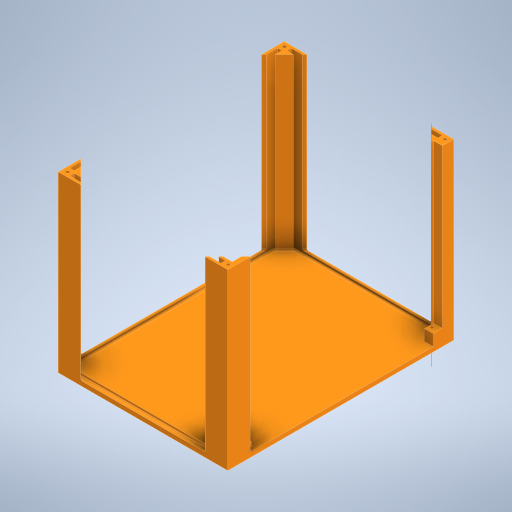
# Autodesk Inventor part: Cabinet
Saved by Autodesk Inventor 2024.3 (Build 283343000, 343)
## iProperties
Created: 2025-03-25
Part Number: Cabinet
Material: Všeobecné
Document SubType Name: Modeling
Designer: admin
Density: 1 g/cm^3
Appearance: Oranžová
Author: admin
Autodesk Inventor part; units mm, degrees
ref_plane "YZ Plane" through (0, 0, 0) normal (1, 0, 0) x (0, 1, 0)
ref_plane "XZ Plane" through (0, 0, 0) normal (0, 1, 0) x (-1, 0, 0)
sketch "Náčrt1" plane through (0, 0, 0) normal (0, 1, 0) x (-1, 0, 0)
  line L0 (75, 100) -> (-75, 100)
  line L1 (-75, 100) -> (-75, -100)
  line L2 (-75, -100) -> (75, -100)
  line L3 (75, -100) -> (75, 100)
  line L4 (105, 0) -> (-105, 0) projected
  line L5 (0, -140) -> (0, 140) projected
  point P0 (0, 0)
  dimension "d0" = 200
  dimension "d1" = 150
  constraints: 8 end point, 2 parallel, 1 horizontal, 1 perpendicular, 2 other
  measures "d0" distance of L2.end L0.start
  measures "d1" distance of L0.start L0.end
extrude "Vysunutí1" add sketch "Náčrt1" along normal blind 4
sketch "Náčrt2" plane through (0, 4, 0) normal (0, 1, 0) x (1, 0, 0)
  line L0 (-75, -100) -> (-75, -80)
  line L1 (-75, -100) -> (-55, -100)
  line L2 (-75, 100) -> (-75, -100) projected
  line L3 (-75, -100) -> (75, -100) projected
  line L4 (-69, -86) -> (-69, -92)
  line L5 (-69, -92) -> (-73, -92)
  line L6 (-73, -92) -> (-73, -82)
  line L7 (-73, -82) -> (-75, -80)
  line L8 (-67, -98) -> (-57, -98)
  line L9 (-61, -94) -> (-67, -94)
  line L10 (-67, -94) -> (-67, -98)
  line L11 (-55, -100) -> (-57, -98)
  line L12 (-61, -94) -> (-69, -86)
  point P0 (0, 0)
  dimension "d4" = 20
  dimension "d9" = 2
  dimension "d10" = 4
  dimension "d11" = 10
  dimension "d12" = 6
  dimension "d13" = 8
  dimension "d17" = 4
  dimension "d18" = 2
  dimension "d19" = 8
  dimension "d20" = 10
  dimension "d21" = 6
  constraints: 22 end point, 2 collinear, 2 horizontal, 2 parallel, 1 perpendicular, 1 vertical
  measures "d4" distance of L0.start L0.end
  measures "d9" distance between parallel lines of L0 L6
  measures "d10" distance of L4.end L5.end
  measures "d11" distance of L5.end L6.end
  measures "d12" distance of L4.start L4.end
  measures "d13" distance between parallel lines of L1 L5
  measures "d17" distance of L9.end L8.start
  measures "d18" distance between parallel lines of L1 L8
  measures "d19" distance between parallel lines of L0 L10
  measures "d20" distance of L8.start L8.end
  measures "d21" distance of L9.start L9.end
extrude "Vysunutí2" add sketch "Náčrt2" along normal blind 150
mirror "Zrcadlit1" about plane through (0, 0, 0) normal (0, 0, 1) of "Vysunutí2"
sketch "Náčrt3" plane through (0, 154, 0) normal (0, 1, 0) x (1, 0, 0)
  line L0 (-69, -92) -> (-73, -92) projected
  line L1 (-67, -98) -> (-67, -94) projected
  point P0 (0, 0)
  point P1 (-71, -96)
  dimension "d22" = 4
  dimension "d23" = 4
  measures "d22" distance from line of point (-71, -96) L0
  measures "d23" distance from line of point (-71, -96) L1
hole "Díra1" at (-71, 154, 96) direction (0, -1, 0) diameter 3 depth 15 tip angle 118
mirror "Zrcadlit2" about plane through (0, 0, 0) normal (0, 0, 1) of "Díra1"
sketch "Náčrt4" plane through (0, 4, 0) normal (0, 1, 0) x (1, 0, 0)
  line L0 (55, -100) -> (75, -100)
  line L1 (75, -100) -> (75, -80)
  line L2 (-55, -100) -> (75, -100) projected
  line L3 (75, -100) -> (75, 100) projected
  line L4 (57, -98) -> (67, -98)
  line L5 (67, -98) -> (67, -94)
  line L6 (67, -94) -> (61, -94)
  line L7 (75, -80) -> (61, -94)
  line L8 (57, -98) -> (55, -100)
  point P0 (0, 0)
  dimension "d31" = 20
  dimension "d32" = 20
  dimension "d37" = 10
  dimension "d38" = 6
  dimension "d39" = 8
  dimension "d40" = 2
  dimension "d41" = 45
  constraints: 14 end point, 2 collinear, 2 horizontal, 2 perpendicular, 1 parallel
  measures "d31" distance of L0.start L0.end
  measures "d32" distance of L0.end L1.end
  measures "d37" distance of L4.start L4.end
  measures "d38" distance of L5.end L6.end
  measures "d39" distance between parallel lines of L1 L5
  measures "d40" distance between parallel lines of L0 L4
  measures "d41" angle of L1 L7
extrude "Vysunutí3" add sketch "Náčrt4" along normal blind 150
mirror "Zrcadlit3" about plane through (0, 0, 0) normal (0, 0, 1) of "Vysunutí3"
ref_plane "Pracovní rovina1" through (0, 14, 0) normal (0, 1, 0) x (1, 0, 0)
sketch "Náčrt7" plane through (0, 4, 0) normal (0, 1, 0) x (1, 0, 0)
  line L0 (66, -80) -> (71, -80)
  line L1 (71, -80) -> (71, -75)
  line L2 (71, -75) -> (66, -75)
  line L3 (66, -75) -> (66, -80)
  line L4 (75, -80) -> (75, 80) projected
  line L5 (55, -100) -> (75, -100) projected
  point P0 (0, 0)
  dimension "d51" = 4
  dimension "d52" = 5
  dimension "d53" = 20
  dimension "d54" = 5
  constraints: 8 end point, 2 parallel, 1 horizontal, 1 perpendicular
  measures "d51" distance between parallel lines of L4 L1
  measures "d52" distance of L2.end L0.start
  measures "d53" distance between parallel lines of L5 L0
  measures "d54" distance of L1.end L2.end
extrude "Vysunutí6" add sketch "Náčrt7" along normal blind 4
mirror "Zrcadlit4" about plane through (0, 0, 0) normal (1, 0, 0) of "Díra1", "Zrcadlit2"
sketch "Náčrt9" plane through (0, 4, 0) normal (0, 1, 0) x (1, 0, 0)
  line L0 (-67, -94) -> (67, -94)
  line L1 (67, -94) -> (67, -98)
  line L2 (67, -98) -> (-67, -98)
  line L3 (-67, -98) -> (-67, -94)
  line L4 (-67, -98) -> (-67, -94) projected
  line L5 (67, -94) -> (67, -98) projected
  line L6 (-57, -98) -> (-67, -98) projected
  line L7 (-67, -94) -> (-61, -94) projected
  point P0 (0, 0)
  constraints: 8 end point, 4 collinear, 2 parallel, 1 horizontal, 1 perpendicular
extrude "Vysunutí7" cut sketch "Náčrt9" against normal blind 2
mirror "Zrcadlit5" about plane through (0, 0, 0) normal (0, 0, 1) of "Vysunutí7"
sketch "Náčrt10" plane through (0, 4, 0) normal (0, 1, 0) x (1, 0, 0)
  line L0 (-69, -92) -> (-73, -92)
  line L1 (-73, -92) -> (-73, 92)
  line L2 (-73, 92) -> (-69, 92)
  line L3 (-69, 92) -> (-69, -92)
  line L4 (-69, 92) -> (-73, 92) projected
  line L5 (-69, -92) -> (-73, -92) projected
  line L6 (-73, -92) -> (-73, -82) projected
  line L7 (-69, -86) -> (-69, -92) projected
  point P0 (0, 0)
  constraints: 8 end point, 4 collinear, 2 parallel, 1 horizontal, 1 perpendicular
extrude "Vysunutí8" cut sketch "Náčrt10" against normal blind 2
sketch "Náčrt11" plane through (0, 154, 0) normal (0, 1, 0) x (1, 0, 0)
  line L0 (63, -92) -> (71, -92)
  line L1 (71, -92) -> (71, -84)
  line L2 (71, -84) -> (63, -84)
  line L3 (63, -84) -> (63, -92)
  line L4 (66, -80) -> (71, -80) projected
  line L5 (75, -80) -> (75, 80) projected
  line L6 (75, -80) -> (61, -94) projected
  point P0 (0, 0)
  dimension "d70" = 8
  dimension "d71" = 4
  constraints: 8 end point, 2 parallel, 2 point on line, 1 horizontal, 1 perpendicular
  measures "d70" distance of L2.end L0.start
  measures "d71" distance between parallel lines of L5 L1
extrude "Vysunutí9" cut sketch "Náčrt11" against normal up to surface (150 mm away)
fillet "Zaoblení1" radius 1 12 edges at (-65, 4, 90) (-56, 4, 99) (-74, 4, 81) (-65, 4, -90) (-74, 4, -81) (-56, 4, -99) (56, 4, -99) (56, 4, 99) (62, 4, 93) (73, 4, 82) (67, 4, 92) (71, 4, 88)
sketch "Náčrt13" plane through (55, 154, -100) normal (0, 1, 0) x (1, 0, 0)
  line L0 (20, -10) -> (12, -10)
  line L1 (12, -10) -> (12, -20)
  line L2 (12, -20) -> (20, -20)
  line L3 (20, -20) -> (20, -10)
  line L4 (20, 0) -> (20, -20) projected
  point P0 (-55, -100)
  dimension "d78" = 10
  dimension "d79" = 8
  constraints: 8 end point, 2 parallel, 1 collinear, 1 horizontal, 1 perpendicular
  measures "d78" distance of L0.end L1.end
  measures "d79" distance of L1.end L2.end
extrude "Vysunutí11" cut sketch "Náčrt13" against normal up to surface (150 mm away)
sketch "Náčrt14" plane through (0, 4, 0) normal (0, 1, 0) x (1, 0, 0)
  line L0 (67, 82) -> (75, 82)
  line L1 (75, 82) -> (75, 90)
  line L2 (75, 90) -> (67, 90)
  line L3 (67, 90) -> (67, 82)
  line L4 (67, 88) -> (67, 90) projected
  line L5 (67, 90) -> (75, 90) projected
  line L6 (75, -78.5858) -> (75, 90) projected
  point P0 (0, 0)
  dimension "d82" = 8
  constraints: 8 end point, 3 collinear, 2 parallel, 1 horizontal, 1 perpendicular
  measures "d82" distance of L0.end L1.end
extrude "Vysunutí12" add sketch "Náčrt14" along normal blind 10
sketch "Náčrt15" plane through (0, 14, 0) normal (0, 1, 0) x (1, 0, 0)
  line L0 (75, 82) -> (75, 90) projected
  line L1 (67, 90) -> (75, 90) projected
  point P0 (0, 0)
  point P1 (69.5, 86)
  dimension "d85" = 5.5
  dimension "d86" = 4
  measures "d85" distance from line of L0 point (69.5, 86)
  measures "d86" distance from line of L1 point (69.5, 86)
hole "Díra3" at (69.5, 14, -86) direction (0, -1, 0) diameter 3 depth 5
